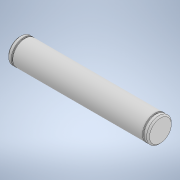
# Autodesk Inventor part: Shatf_piston
Saved by Autodesk Inventor 2022 (Build 260153000, 153)
## iProperties
Created: 2022-04-09
Part Number: Shatf_piston
Material: Generic
Document SubType Name: Modeling
Designer: Patrick
Density: 1 g/cm^3
Appearance: Default
Author: Patrick
Autodesk Inventor part; units mm, degrees
ref_plane "YZ Plane" through (0, 0, 0) normal (1, 0, 0) x (0, 1, 0)
ref_plane "XZ Plane" through (0, 0, 0) normal (0, 1, 0) x (-1, 0, 0)
ref_plane "XY Plane" through (0, 0, 0) normal (0, 0, 1) x (1, 0, 0)
sketch "Sketch1" plane through (0, 0, 0) normal (0, 1, 0) x (-1, 0, 0)
  line L0 (0, 0) -> (0, -5.2929)
  line L1 (0, -5.2929) -> (-0.7071, -6)
  line L2 (-0.7071, -6) -> (-2, -6)
  line L3 (-2, -6) -> (-2, -5.5)
  line L4 (-2, -5.5) -> (-2.7, -5.5)
  line L5 (-2.7, -5.5) -> (-2.7, -6)
  line L6 (-2.7, -6) -> (-34.2, -6)
  line L7 (-34.2, -6) -> (-34.2, 0)
  line L8 (-34.2, 0) -> (0, 0)
  line L9 (-68.4, 0) -> (-68.4, -5.2929)
  line L10 (-68.4, -5.2929) -> (-67.6929, -6)
  line L11 (-67.6929, -6) -> (-66.4, -6)
  line L12 (-66.4, -6) -> (-66.4, -5.5)
  line L13 (-66.4, -5.5) -> (-65.7, -5.5)
  line L14 (-65.7, -5.5) -> (-65.7, -6)
  line L15 (-65.7, -6) -> (-34.2, -6)
  line L16 (-68.4, 0) -> (-34.2, 0)
  dimension "d0" = 6
  dimension "d1" = 0.7
  dimension "d2" = 2
  dimension "d3" = 0.5
  dimension "d4" = 135
  dimension "d5" = 1
  dimension "d8" = 31.5
  constraints: 34 end point, 7 symmetric about line, 6 perpendicular, 4 point on line, 1 horizontal, 1 vertical
  measures "d0" distance between parallel lines of L8 L6
  measures "d1" distance between parallel lines of L5 L3
  measures "d2" distance between parallel lines of L3 L0
  measures "d3" distance from line of L1.end L4
  measures "d4" angle of L0 L1
  measures "d5" distance of L0.end L1.end
  measures "d8" distance between parallel lines of L7 L5
revolve "Revolution1" add sketch "Sketch1" angle 360 about axis through (68.4, 0, 0) along (-1, 0, 0)
body "Solid1"
